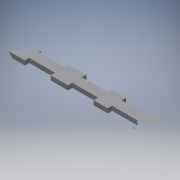
# Autodesk Inventor part: top
Saved by Autodesk Inventor 2016 (Build 200138000, 138)
## iProperties
Created: 2016-05-17
Part Number: top
Material: Generic
Document SubType Name: Modeling
Designer: Lillahunden
Density: 1 g/cm^3
Appearance: Default
Author: Lillahunden
Autodesk Inventor part; units mm, degrees
ref_plane "YZ Plane" through (0, 0, 0) normal (1, 0, 0) x (0, 1, 0)
ref_plane "XZ Plane" through (0, 0, 0) normal (0, 1, 0) x (-1, 0, 0)
ref_plane "XY Plane" through (0, 0, 0) normal (0, 0, 1) x (1, 0, 0)
sketch "Sketch1" plane through (0, 0, 0) normal (0, 0, 1) x (1, 0, 0)
  line L0 (200, 0) -> (171.6283, 0) construction
  line L1 (200, 6) -> (200, 0)
  line L2 (171.6283, 6) -> (200, 6)
  line L3 (171.6283, 6) -> (171.6283, 0)
  line L4 (136.6283, 6) -> (136.6283, 0)
  line L5 (136.6283, 0) -> (171.6283, 0)
  line L6 (171.6283, 0) -> (171.6283, 6)
  line L7 (136.6283, 6) -> (171.6283, 6)
  line L8 (136.6283, 0) -> (117.5, 0) construction
  line L9 (136.6283, 6) -> (136.6283, 0)
  line L10 (117.5, 6) -> (136.6283, 6)
  line L11 (117.5, 6) -> (117.5, 0)
  line L12 (117.5, 0) -> (117.5, 6)
  line L13 (82.5, 6) -> (117.5, 6)
  line L14 (82.5, 6) -> (82.5, 0)
  line L15 (82.5, 0) -> (117.5, 0)
  line L16 (82.5, 0) -> (58.75, 0) construction
  line L17 (82.5, 6) -> (82.5, 0)
  line L18 (58.75, 6) -> (82.5, 6)
  line L19 (58.75, 6) -> (58.75, 0)
  line L20 (23.75, 6) -> (23.75, 0)
  line L21 (23.75, 0) -> (58.75, 0)
  line L22 (58.75, 0) -> (58.75, 6)
  line L23 (23.75, 6) -> (58.75, 6)
  line L24 (23.75, 0) -> (0, 0) construction
  line L25 (23.75, 6) -> (23.75, 0)
  line L26 (0, 6) -> (23.75, 6)
  line L27 (0, 0) -> (0, 6)
  line L28 (200, 6) -> (1.5061, 6)
  line L29 (1.5061, 6) -> (1.5061, -19)
  line L30 (1.5061, -19) -> (200, -19)
  line L31 (200, -19) -> (200, 6)
extrude "Extrusion1" add sketch "Sketch1" against normal blind 6 contours L1 L31 L30 L29 L26 L20 L21 L19 L18 L14 L15 L11 L10 L4 L5 L3 L2
sketch "Sketch2" plane through (0, 0, 0) normal (0, 0, 1) x (1, 0, 0)
  line L0 (200, 6) -> (171.6283, 6) projected
  line L1 (171.6283, 0) -> (171.6283, 6) projected
  line L2 (136.6283, 0) -> (171.6283, 0) projected
  line L3 (136.6283, 6) -> (136.6283, 0) projected
  line L4 (136.6283, 6) -> (117.5, 6) projected
  line L5 (117.5, 0) -> (82.5, 0) projected
  line L6 (82.5, 6) -> (82.5, 0) projected
  line L7 (82.5, 6) -> (58.75, 6) projected
  line L8 (58.75, 0) -> (58.75, 6) projected
  line L9 (58.75, 0) -> (23.75, 0) projected
  line L10 (23.75, 0) -> (23.75, 6) projected
  line L11 (23.75, 6) -> (1.5061, 6) projected
  line L12 (1.5061, -19) -> (200, -19) construction
  line L13 (200, -19) -> (1.5061, -19) construction
  line L14 (195.1496, -19) -> (195.1496, 6) construction
  line L15 (171.6283, 6) -> (200, 6) construction
  line L16 (195.1496, -6.5) -> (183.8978, -6.5) construction
  line L17 (200, -19) -> (171.6283, -19)
  line L18 (171.6283, -13) -> (171.6283, -19)
  line L19 (136.6283, -13) -> (171.6283, -13)
  line L20 (136.6283, -19) -> (136.6283, -13)
  line L21 (136.6283, -19) -> (117.5, -19)
  line L22 (117.5, -13) -> (82.5, -13)
  line L23 (82.5, -19) -> (82.5, -13)
  line L24 (82.5, -19) -> (58.75, -19)
  line L25 (58.75, -13) -> (58.75, -19)
  line L26 (58.75, -13) -> (23.75, -13)
  line L27 (23.75, -13) -> (23.75, -19)
  line L28 (23.75, -19) -> (1.5061, -19)
  line L29 (195.1496, 6) -> (195.1496, -19) construction
  line L30 (171.6283, -19) -> (200, -19) construction
  line L31 (117.5, -13) -> (117.5, -19)
  line L32 (82.5, -19) -> (117.5, -19)
  line L33 (23.75, -19) -> (58.75, -19)
  line L34 (171.6283, -19) -> (136.6283, -19)
  point P0 (0, 0)
  point P1 (0, -13)
  constraints: 30 end point, 15 symmetric about line, 3 collinear, 3 point on line, 2 perpendicular, 1 horizontal, 1 midpoint
extrude "Extrusion2" cut sketch "Sketch2" against normal through all
move faces "Move1" translate (-1.5061, 0, 0) faces at (1.5061, -2.3333, -2)
body "Solid1"
